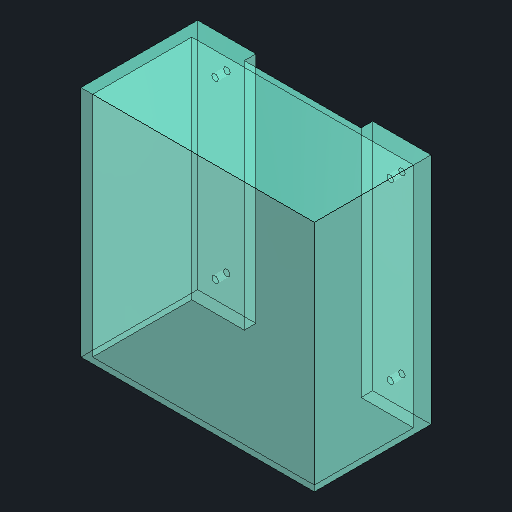
# Autodesk Inventor part: KN-00-00-01
Saved by Autodesk Inventor 2025.2 (Build 292293000, 293)
## iProperties
Created: 2025-04-28
Part Number: KN-00-00-01
Material: PET Plastic
Document SubType Name: Modeling
Designer: Kacper Mik
Density: 1.541 g/cm^3
Appearance: Indoor Pool
Author: Kacper Mik
Autodesk Inventor part; units mm, degrees
ref_plane "YZ Plane" through (0, 0, 0) normal (1, 0, 0) x (0, 1, 0)
ref_plane "XZ Plane" through (0, 0, 0) normal (0, 1, 0) x (-1, 0, 0)
ref_plane "XY Plane" through (0, 0, 0) normal (0, 0, 1) x (1, 0, 0)
sketch "Sketch3" plane through (0, 0, 0) normal (0, 0, 1) x (1, 0, 0)
  line L0 (-100, -100) -> (100, -100)
  line L1 (100, -100) -> (100, 100)
  line L2 (100, 100) -> (-100, 100)
  line L3 (-100, 100) -> (-100, -100)
  line L4 (-100, -100) -> (100, 100) construction
  line L5 (100, -100) -> (-100, 100) construction
  point P0 (0, 0)
  dimension "d8" = 200
  dimension "d9" = 200
  constraints: 12 end point, 2 midpoint, 2 parallel, 1 horizontal, 1 perpendicular
  measures "d8" distance of L1.end L2.end
  measures "d9" distance of L2.end L0.start
extrude "Extrusion2" add sketch "Sketch3" along normal blind 90
shell "Shell2" thickness 5 removed faces 2 at (-33.3333, -100, 30) at (-33.3333, -33.3333, 0)
sketch "Sketch4" plane through (0, 0, 0) normal (0, 0, 1) x (1, 0, 0)
  line L0 (100, -100) -> (100, 100) construction
  line L1 (100, 100) -> (-100, 100) construction
  line L2 (-100, 100) -> (-100, -100) construction
  line L3 (-100, -100) -> (100, -100) construction
  line L4 (-100, 100) -> (100, 100)
  line L5 (100, 100) -> (100, -100)
  line L6 (-100, -100) -> (-100, 100)
  line L7 (0, -140) -> (0, 140) projected
  point P0 (0, 0)
  point P1 (-75, -75)
  point P2 (75, -75)
  point P3 (-75, 75)
  point P4 (75, 75)
  dimension "d13" = 150
  dimension "d14" = 25
  dimension "d15" = 150
  constraints: 6 end point, 2 horizontal alignment, 2 vertical alignment, 1 horizontal, 1 parallel, 1 perpendicular, 1 symmetric about line
  measures "d13" distance of point (-75, -75) point (-75, 75)
  measures "d14" distance from line of L3 point (-75, -75)
  measures "d15" distance of point (75, -75) point (-75, -75)
sketch "Sketch5" plane through (0, 0, 0) normal (0, 0, 1) x (1, 0, 0)
  line L0 (-100, 100) -> (-100, -100) projected
  line L1 (100, 100) -> (-100, 100)
  line L2 (-100, 100) -> (-100, -100)
  line L3 (100, -100) -> (100, 100)
  line L4 (-100, -100) -> (100, -100) projected
  line L5 (100, -100) -> (50, -100)
  line L6 (50, -100) -> (50, 100)
  line L7 (-50, -100) -> (-50, 100)
  point P0 (0, 0)
  dimension "d16" = 50
  dimension "d17" = 50
  constraints: 12 end point, 4 point on line, 3 perpendicular, 1 horizontal, 1 parallel
  measures "d16" distance of L3.start L5.end
  measures "d17" distance between parallel lines of L0 L7
extrude "Extrusion3" add sketch "Sketch5" against normal blind 10 contours L1 L7 L4 L0 | L1 L3 L4 L6
hole "Hole1" at (-75, -75, 0) at (75, -75, 0) at (-75, 75, 0) at (75, 75, 0) direction (0, 0, -1) diameter 5.5 end through all clearance for "Countersunk Flat Head Screw ISO 2009/7046" size "M5" standard "ISO"
equation "\"d17\" = d16"
body "Solid2"
